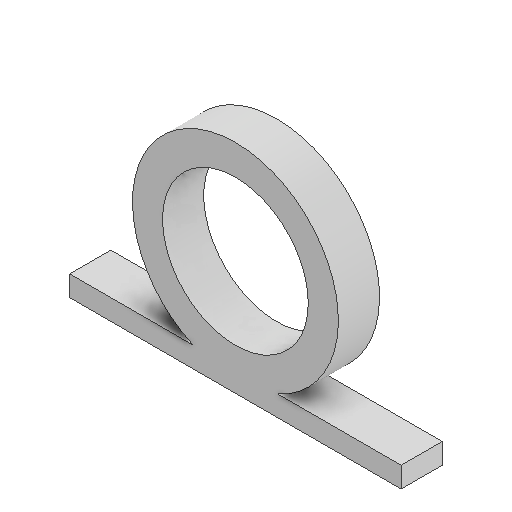
# Autodesk Inventor part: d35_hole
Saved by Autodesk Inventor 2026.2 (Build 302298000, 298)
## iProperties
Created: 2026-06-18
Part Number: d35_hole
Material: Generic
Document SubType Name: Modeling
Designer: zetsu
Density: 1 g/cm^3
Appearance: Default
Author: zetsu
Autodesk Inventor part; units mm, degrees
ref_plane "YZ Plane" through (0, 0, 0) normal (1, 0, 0) x (0, 1, 0)
ref_plane "XZ Plane" through (0, 0, 0) normal (0, 1, 0) x (-1, 0, 0)
ref_plane "XY Plane" through (0, 0, 0) normal (0, 0, 1) x (1, 0, 0)
sketch "スケッチ1" plane through (0, 0, 0) normal (0, 0, 1) x (1, 0, 0)
  circle A0 centre (0, 0) radius 17.7
  arc A1 (10.2674, -22.7943) -> (-10.2674, -22.7943) centre (0, 0) ccw
  line L0 (-10.2674, -22.7943) -> (-40.2674, -22.7943)
  line L1 (-40.2674, -22.7943) -> (-40.2674, -27.7943)
  line L2 (10.2674, -22.7943) -> (40.2674, -22.7943)
  line L3 (40.2674, -22.7943) -> (40.2674, -27.7943)
  line L4 (40.2674, -27.7943) -> (-40.2674, -27.7943)
  dimension "d0" = 35.4
  dimension "d1" = 25
  dimension "d2" = 30
  dimension "d3" = 5
  dimension "d4" = 30
  dimension "d5" = 5
  constraints: 10 end point, 3 perpendicular, 2 centre point, 2 coincident, 2 horizontal, 2 point on circle
  measures "d0" diameter of A0
  measures "d1" radius of A1
  measures "d2" distance of L0.start L0.end
  measures "d3" distance of L0.end L1.end
  measures "d4" distance of L2.start L2.end
  measures "d5" distance of L2.end L3.end
extrude "押し出し1" add sketch "スケッチ1" along normal blind 10
